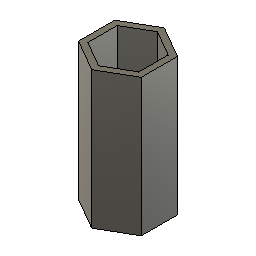
hexagon-02 (Autodesk Fusion 360 design; units mm, degrees)
Autodesk Fusion 360 part; units mm, degrees
sketch "Sketch1" plane through (0, 0, 0) normal (0, 1, 0) x (1, 0, 0)
  line L0 (16, 9.2376) -> (0, 18.4752)
  line L1 (0, 18.4752) -> (-16, 9.2376)
  line L2 (-16, 9.2376) -> (-16, -9.2376)
  line L3 (-16, -9.2376) -> (0, -18.4752)
  line L4 (0, -18.4752) -> (16, -9.2376)
  line L5 (16, -9.2376) -> (16, 9.2376)
  line L6 (13, 7.5056) -> (0, 15.0111)
  line L7 (0, 15.0111) -> (-13, 7.5056)
  line L8 (-13, 7.5056) -> (-13, -7.5056)
  line L9 (-13, -7.5056) -> (0, -15.0111)
  line L10 (0, -15.0111) -> (13, -7.5056)
  line L11 (13, -7.5056) -> (13, 7.5056)
  dimension "d1" = 16
  dimension "d2" = 3
  measures "d1" distance of origin L5
  measures "d2" distance of L5 L11
extrude "Extrude1" add sketch "Sketch1" along normal blind 70 makes body 1
extrude "Extrude2" add sketch "Sketch1" along normal blind 3 contours L6 L7 L8 L9 L10 L11 bodies 1
copy_body "Body->Comp1" bodies 1 removing the originals makes body 2 in component "hexagon-02"
component "hexagon-02" placed x (1, 0, 0) y (0, 1, 0) z (0, 0, 1) at (0, 0, 0)
